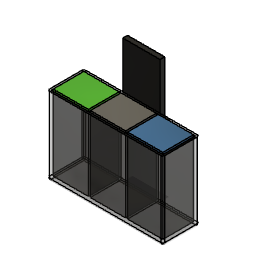
Incubator v2 (Autodesk Fusion 360 design; units mm, degrees)
Autodesk Fusion 360 part; units mm, degrees
sketch "Sketch1" plane through (0, 0, 0) normal (0, 1, 0) x (1, 0, 0)
  line L0 (-55, 25) -> (65, 25)
  line L1 (65, 25) -> (65, -10)
  line L2 (65, -10) -> (-55, -10)
  line L3 (-55, -10) -> (-55, 25)
  line L4 (-55, 25) -> (-15, 25)
  line L5 (-15, -10) -> (-55, -10)
  line L6 (-55, -10) -> (-55, 25)
  line L7 (-15, 25) -> (25, 25)
  line L8 (25, -10) -> (-15, -10)
  line L9 (-57, 27) -> (67, 27)
  line L10 (67, 27) -> (67, -12)
  line L11 (67, -12) -> (-57, -12)
  line L12 (-57, -12) -> (-57, 27)
  line L13 (-14, 24) -> (24, 24)
  line L14 (24, 24) -> (24, -9)
  line L15 (24, -9) -> (-14, -9)
  line L16 (-14, -9) -> (-14, 24)
  line L17 (-16, 24) -> (-16, -9)
  line L18 (-16, -9) -> (-54, -9)
  line L19 (-54, -9) -> (-54, 24)
  line L20 (-54, 24) -> (-16, 24)
  line L21 (-16, -9) -> (-16, 24)
  line L22 (64, 24) -> (64, -9)
  line L23 (-54, -9) -> (-54, 24)
  line L24 (26, 24) -> (26, -9)
  line L25 (-54, 24) -> (-16, 24)
  line L26 (-16, -9) -> (-54, -9)
  line L27 (64, -9) -> (26, -9)
  line L28 (24, -9) -> (-14, -9)
  line L29 (-14, 24) -> (24, 24)
  line L30 (26, 24) -> (64, 24)
  dimension "d1" = 120
  dimension "d2" = 35
  dimension "d3" = 40
  dimension "d4" = 40
  dimension "d5" = -2
  constraint horizontal L0
  constraint vertical L1
  constraint horizontal L2
  constraint vertical L3
  constraint horizontal L4
  constraint horizontal L5
  constraint vertical L6
  constraint horizontal L7
  constraint horizontal L8
  constraint coincident L24.start L25
  constraint collinear L25 L29
  constraint collinear L26 L27
  constraint collinear L27 L28
  constraint collinear L29 L30
  measures "d1" distance of L0.start L0.end
  measures "d2" distance of L0.start L2.end
  measures "d3" distance of L0.start L4.end
  measures "d4" distance of L4.end L7.end
extrude "Extrude1" add sketch "Sketch1" along normal blind 80 contours L9 L10 L11 L12 makes body 1
extrude "Extrude2" add sketch "Sketch1" along normal blind 79 contours L0 L1 L2 L3 L4 L5 L6 L7 L8 bodies 1
sketch "Sketch2" plane through (0, 79, 0) normal (0, 1, 0) x (-1, 0, 0)
  line L0 (14, 9) -> (14, -24)
  line L1 (14, -24) -> (-24, -24)
  line L2 (-24, -24) -> (-24, 9)
  line L3 (-24, 9) -> (14, 9)
  line L4 (16, -24) -> (16, 9)
  line L5 (16, 9) -> (54, 9)
  line L6 (54, 9) -> (54, -24)
  line L7 (54, -24) -> (16, -24)
  line L8 (-26, 9) -> (-26, -24)
  line L9 (-26, -24) -> (-64, -24)
  line L10 (-64, -24) -> (-64, 9)
  line L11 (-64, 9) -> (-26, 9)
  line L12 (55, 10) -> (-65, 10)
  line L13 (-65, 10) -> (-65, -25)
  line L14 (-65, -25) -> (55, -25)
  line L15 (55, -25) -> (55, 10)
  line L16 (55, -25) -> (15, -25)
  line L17 (15, -25) -> (15, 9)
  line L18 (15, 9) -> (55, 9)
  line L19 (55, 9) -> (55, -25)
  constraint horizontal L16
  constraint vertical L17
  constraint horizontal L18
  constraint vertical L19
  constraint coincident L14.end L15.start
extrude "Extrude3" add sketch "Sketch2" along normal blind 2 separate body contours L4 L5 L6 L7 L18 makes body 2
copy_body "CopyPasteBodies1" bodies 2 makes body 3
move_body "Move1" bodies 3 to x (1, 0, 0) y (0, 1, 0) z (0, 0, 1) at (40, 0, 0)
copy_body "CopyPasteBodies2" bodies 2 makes body 4
move_body "Move2" bodies 4 to x (1, 0, 0) y (0, 1, 0) z (0, 0, 1) at (80, 0, 0)
sketch "Sketch3" plane through (0, 0, 0) normal (0, -1, 0) x (1, 0, 0)
  line L0 (26, -24) -> (26, 9)
  line L1 (26, 9) -> (64, 9)
  line L2 (64, 9) -> (64, -24)
  line L3 (64, -24) -> (26, -24)
  line L4 (-16, 9) -> (-16, -24)
  line L5 (-16, -24) -> (-54, -24)
  line L6 (-54, -24) -> (-54, 9)
  line L7 (-54, 9) -> (-16, 9)
  line L8 (-14, -24) -> (-14, 9)
  line L9 (-14, 9) -> (24, 9)
  line L10 (24, 9) -> (24, -24)
  line L11 (24, -24) -> (-14, -24)
  line L12 (67, 12) -> (-57, 12)
  line L13 (-57, 12) -> (-57, -27)
  line L14 (-57, -27) -> (67, -27)
  line L15 (67, -27) -> (67, 12)
  line L16 (-57, 12) -> (67, 12)
  line L17 (67, 12) -> (67, -27)
  line L18 (67, -27) -> (-57, -27)
  line L19 (-57, -27) -> (-57, 12)
  constraint horizontal L16
  constraint vertical L17
  constraint horizontal L18
  constraint vertical L19
  constraint coincident L14.end L15.start
  constraint coincident L12.end L13.start
extrude "Extrude4" add sketch "Sketch3" along normal blind 3 contours L0 L1 L2 L3 | L4 L5 L6 L7 | L8 L9 L10 L11 | L12 L13 L14 L15 L16 L17 L18 L19 bodies 1
sketch "Sketch4" plane through (0, 0, -27) normal (0, 0, -1) x (-1, 0, 0)
  line L0 (57, -3) -> (57, 80)
  line L1 (57, 80) -> (-67, 80)
  line L2 (-67, 80) -> (-67, -3)
  line L3 (-67, -3) -> (57, -3)
  line L4 (-25, 70) -> (15, 70)
  line L5 (15, 70) -> (15, 50)
  line L6 (15, 50) -> (-25, 50)
  line L7 (-25, 50) -> (-25, 70)
  constraint horizontal L4
  constraint vertical L5
  constraint horizontal L6
  constraint vertical L7
extrude "Extrude5" add sketch "Sketch4" along normal blind 10 contours L4 L5 L6 L7 bodies 1
sketch "Sketch5" plane through (0, 70, 0) normal (0, 1, 0) x (-1, 0, 0)
  line L0 (15, -27) -> (-25, -27)
  line L1 (-25, -27) -> (-25, -37)
  line L2 (-25, -37) -> (15, -37)
  line L3 (15, -37) -> (15, -27)
  line L4 (-25, -27) -> (15, -27)
  line L5 (15, -27) -> (15, -32)
  line L6 (15, -32) -> (-25, -32)
  line L7 (-25, -32) -> (-25, -27)
  constraint horizontal L4
  constraint vertical L5
  constraint horizontal L6
  constraint vertical L7
  constraint midpoint L3 L5.end
  constraint coincident L0.end L1.start
extrude "Extrude6" add sketch "Sketch5" along normal blind 60 contours L0 L1 L3 L4 L5 L6 L7 bodies 1
split "Split1" by plane through (-57, 0, -27) normal (0, 0, -1) bodies 1 makes body 5 at (-1.6667, 90, -32)
split "Split2" by plane through (25, 70, -27) normal (0, 1, 0) bodies 5 makes body 6 at (-1.6667, 90, -32)
fillet "Fillet1" radius 2 8 edges at (67, 38.5, 12) (5, -3, 12) (-57, 38.5, 12) (-57, 38.5, -27) (-57, -3, -7.5) (67, 38.5, -27) (5, -3, -27) (67, -3, -7.5) on bodies 1
